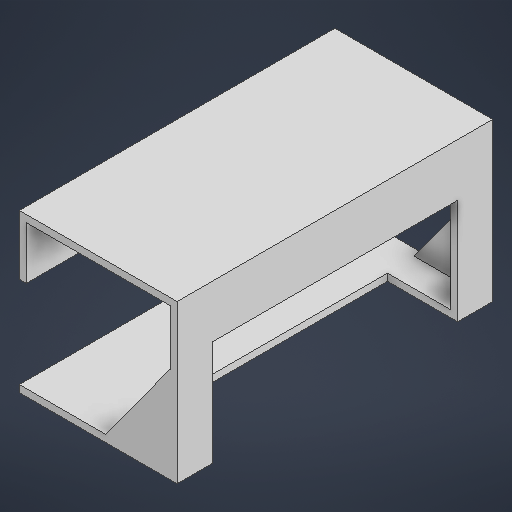
# Autodesk Inventor part: belt_holder
Saved by Autodesk Inventor 2026 (Build 300175000, 175)
## iProperties
Created: 2025-07-15
Part Number: belt_holder
Material: Generic
Document SubType Name: Modeling
Designer: user
Density: 1 g/cm^3
Appearance: Default
Author: user
Autodesk Inventor part; units mm, degrees
ref_plane "YZ Plane" through (0, 0, 0) normal (1, 0, 0) x (0, 1, 0)
ref_plane "XZ Plane" through (0, 0, 0) normal (0, 1, 0) x (-1, 0, 0)
ref_plane "XY Plane" through (0, 0, 0) normal (0, 0, 1) x (1, 0, 0)
sketch "Sketch1" plane through (0, 0, 0) normal (0, 0, 1) x (1, 0, 0)
  line L0 (0, 0) -> (-45, 0)
  line L1 (-45, 0) -> (-45, 45)
  line L2 (-45, 45) -> (0, 45)
  line L3 (0, 45) -> (0, 0)
  line L4 (-2, 45) -> (-2, 0)
  line L5 (-45, 2) -> (-2, 2)
  line L6 (-2, 45) -> (-45, 45)
  line L7 (-45, 45) -> (-45, 43)
  line L8 (-45, 43) -> (-2, 43)
  line L9 (-2, 43) -> (-2, 45)
  line L10 (-45, 43) -> (-43, 43)
  line L11 (-43, 43) -> (-43, 28)
  line L12 (-43, 28) -> (-45, 28)
  line L13 (-45, 28) -> (-45, 43)
  dimension "d0" = 45
  dimension "d1" = 45
  dimension "d2" = 2
  dimension "d3" = 2
  dimension "d17" = 2
  dimension "d18" = 2
  dimension "d19" = 15
  constraints: 28 end point, 6 parallel, 5 perpendicular, 5 point on line, 3 horizontal
  measures "d0" distance of L1.end L2.end
  measures "d1" distance of L0.end L1.end
  measures "d2" distance between parallel lines of L3 L4
  measures "d3" distance between parallel lines of L5 L0
  measures "d17" distance of L7.end L6.end
  measures "d18" distance of L11.end L12.end
  measures "d19" distance of L10.end L11.end
extrude "Extrusion1" add sketch "Sketch1" along normal blind 90 contours L0 L4 L2 L3 | L0 L1 L5 L4
sketch "Sketch2" plane through (0, 0, 90) normal (0, 0, 1) x (1, 0, 0)
  line L0 (-45, 0) -> (0, 0) projected
  line L1 (0, 0) -> (-30, 0)
  line L2 (-30, 0) -> (-30, 30)
  line L3 (-30, 30) -> (0, 30)
  line L4 (0, 30) -> (0, 0)
  line L5 (0, 0) -> (-21.8882, 0)
  line L6 (-21.8882, 0) -> (0, 30)
  dimension "d6" = 30
  dimension "d7" = 30
  dimension "d8" = 30
  constraints: 12 end point, 2 parallel, 2 perpendicular, 2 point on line, 1 horizontal
  measures "d6" distance of L2.end L3.end
  measures "d7" distance of L1.end L2.end
  measures "d8" distance of L0.end L6.end
extrude "Extrusion2" add sketch "Sketch2" against normal blind 2 contours L6 L4 L0
ref_plane "Work Plane1" through (0, 0, 45) normal (0, 0, -1) x (-1, 0, 0)
mirror "Mirror1" about plane through (0, 0, 45) normal (0, 0, -1) of "Extrusion2"
sketch "Sketch3" plane through (0, 0, 0) normal (1, 0, 0) x (0, 0, -1)
  line L0 (-80, 30) -> (-10, 30)
  line L1 (-10, 30) -> (-10, -10)
  line L2 (-10, -10) -> (-80, -10)
  line L3 (-80, -10) -> (-80, 30)
  line L4 (0, 45) -> (-90, 45) projected
  line L5 (0, 0) -> (0, 45) projected
  dimension "d11" = 70
  dimension "d12" = 40
  dimension "d13" = 15
  dimension "d14" = 10
  constraints: 8 end point, 2 parallel, 1 horizontal, 1 perpendicular
  measures "d11" distance of L1.end L2.end
  measures "d12" distance of L0.end L1.end
  measures "d13" distance between parallel lines of L4 L0
  measures "d14" distance between parallel lines of L5 L1
extrude "Extrusion3" cut sketch "Sketch3" against normal blind 20
extrude "Extrusion4" add sketch "Sketch1" along normal blind 90 contours L4 L8 L1 L2 | L1 L8 L11 L12
body "Solid1"
